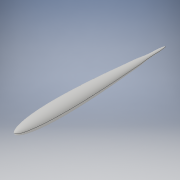
# Autodesk Inventor part: fuselage
Saved by Autodesk Inventor 2019 (Build 230136000, 136)
## iProperties
Created: 2019-04-06
Part Number: fuselage
Material: Generic
Document SubType Name: Modeling
Designer: albaa
Density: 1 g/cm^3
Appearance: Default
Author: albaa
Autodesk Inventor part; units mm, degrees
ref_plane "YZ Plane" through (0, 0, 0) normal (1, 0, 0) x (0, 1, 0)
ref_plane "XZ Plane" through (0, 0, 0) normal (0, 1, 0) x (-1, 0, 0)
ref_plane "XY Plane" through (0, 0, 0) normal (0, 0, 1) x (1, 0, 0)
sketch "Sketch1" plane through (0, 0, 0) normal (0, 1, 0) x (-1, 0, 0)
  spline S0 degree 5 poles (1.89, -2000) (7.719258, -1992.797092) (15.942458, -1933.60907) (17.869846, -1739.851125) (36.745642, -1701.073562) (46.1191, -1490.996356) (59.028641, -1360.902903) (68.511539, -1199.039495) (77.213925, -1054.911349) (83.625866, -912.398524) (88.123661, -779.187766) (90.325519, -653.584973) (90.314427, -537.462975) (87.88304, -431.1689) (83.448701, -335.721413) (76.56647, -251.409033) (68.541618, -179.323734) (57.896886, -118.875494) (47.627633, -71.280296) (33.744189, -33.770014) (21.096578, -8.508569) (0, 7.046704) (-21.096578, -8.508569) (-33.744189, -33.770014) (-47.627634, -71.280296) (-57.89688, -118.875493) (-68.541638, -179.323735) (-76.566403, -251.409027) (-83.448914, -335.72143) (-87.882393, -431.168848) (-90.316312, -537.463125) (-90.320214, -653.584551) (-88.138159, -779.18892) (-83.587223, -912.395449) (-77.31467, -1054.919367) (-68.254061, -1199.019004) (-59.674819, -1360.954325) (-44.519204, -1491.718928) (-40.776152, -1679.630047) (-14.632375, -1736.329849) (-19.682396, -1918.394752) (-8.449579, -1994.057196) (-1.471241, -2004.153309) (1.89, -2000) knots 0 0 0 0 0 0 0.040547 0.0674151 0.10081985 0.13386281 0.16642628 0.19839026 0.22963211 0.26002603 0.28944214 0.31774511 0.3447921 0.37042968 0.39448947 0.41678231 0.43709234 0.4551844 0.47092536 0.48470486 0.49744247 0.51018008 0.52395958 0.53970054 0.5577926 0.57810263 0.60039547 0.62445526 0.65009284 0.67713983 0.7054428 0.73485891 0.76525283 0.79649469 0.82845867 0.86102213 0.89406509 0.92746984 0.95536096 0.97661997 1 1 1 1 1 1
  line L0 (0, 0) -> (0, -2001.13658)
  line L1 (0, -2436.71126) -> (0, 477.03289)
  point P0 (15.225378, -6.831014)
  point P1 (29.60123, -27.277393)
  point P2 (42.983401, -61.199468)
  point P3 (55.165573, -108.365517)
  point P4 (65.901354, -168.453347)
  point P5 (74.931246, -241.052498)
  point P6 (82.011122, -325.667043)
  point P7 (86.938641, -421.718981)
  point P8 (89.574226, -528.552179)
  point P9 (89.853891, -645.436857)
  point P10 (87.792168, -771.574575)
  point P11 (83.47462, -906.103684)
  point P12 (77.04071, -1048.105214)
  point P13 (68.659106, -1196.609151)
  point P14 (58.498468, -1350.601062)
  point P15 (46.697567, -1509.029026)
  point P16 (33.338768, -1670.810819)
  point P17 (-15.225378, -6.831014)
  point P18 (-29.60123, -27.277393)
  point P19 (-42.983401, -61.199468)
  point P20 (-55.165573, -108.365517)
  point P21 (-65.901354, -168.453347)
  point P22 (-74.931246, -241.052498)
  point P23 (-82.011122, -325.667043)
  point P24 (-86.938641, -421.718981)
  point P25 (-89.574226, -528.552179)
  point P26 (-89.853891, -645.436857)
  point P27 (-87.792168, -771.574575)
  point P28 (-83.47462, -906.103684)
  point P29 (-77.04071, -1048.105214)
  point P30 (-68.659106, -1196.609151)
  point P31 (-58.498468, -1350.601062)
  point P32 (-46.697567, -1509.029026)
  point P33 (-33.338768, -1670.810819)
  point P34 (-18.4288, -1834.841309)
  point P35 (-1.89, -2000)
  constraints: 2 end point, 1 vertical, 81 other
revolve "Revolution1" add sketch "Sketch1" angle 360 about axis through (0, 0, -10) along (0, 0, 1) picked at (-6.395446, -1272.349072) contours L0 S0
body "Solid1"
